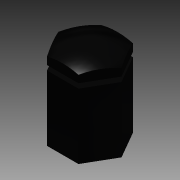
# Autodesk Inventor part: Tapón tornillo
Saved by Autodesk Inventor 2014 (Build 180170000, 170)
## iProperties
Created: 2015-05-28
Part Number: Tapón tornillo
Material: Generic
Document SubType Name: Modeling
Designer: Rubén
Density: 1 g/cm^3
Appearance: Smooth - Black
Author: Rubén
Autodesk Inventor part; units mm, degrees
ref_plane "YZ Plane" through (0, 0, 0) normal (1, 0, 0) x (0, 1, 0)
sketch "Sketch1" plane through (0, 0, 0) normal (0, 1, 0) x (-1, 0, 0)
  circle A0 centre (0, 0) radius 10.25 construction
  line L0 (5.9178, 10.25) -> (11.8357, 0)
  line L1 (11.8357, 0) -> (5.9178, -10.25)
  line L2 (5.9178, -10.25) -> (-5.9178, -10.25)
  line L3 (-5.9178, -10.25) -> (-11.8357, 0)
  line L4 (-11.8357, 0) -> (-5.9178, 10.25)
  line L5 (-5.9178, 10.25) -> (5.9178, 10.25)
  line L6 (0, 0) -> (13.5662, 0) construction
  point P0 (0, 10.25)
  dimension "d1" = 20.5
  constraints: 14 end point, 2 coincident, 1 horizontal, 1 midpoint, 1 parallel, 1 vertical alignment, 15 other
extrude "Extrusion1" add sketch "Sketch1" along normal blind 32
ref_plane "Work Plane1" through (0, 24.5, 0) normal (0, -1, 0) x (1, 0, 0)
sketch "Sketch2" plane through (0, 24.5, 0) normal (0, -1, 0) x (1, 0, 0)
  circle A0 centre (0, 0) radius 7.5 construction
  line L0 (-4.3301, 7.5) -> (4.3301, 7.5)
  line L1 (4.3301, 7.5) -> (8.6603, 0)
  line L2 (8.6603, 0) -> (4.3301, -7.5)
  line L3 (4.3301, -7.5) -> (-4.3301, -7.5)
  line L4 (-4.3301, -7.5) -> (-8.6603, 0)
  line L5 (-8.6603, 0) -> (-4.3301, 7.5)
  line L6 (0, 0) -> (-12.4427, 0) construction
  circle A1 centre (0, 0) radius 12.5
  point P0 (-6.4952, 3.75)
  dimension "d5" = 15
  dimension "d6" = 25
  constraints: 14 end point, 3 coincident, 1 centre point, 1 horizontal, 1 midpoint, 1 parallel, 16 other
  measures "d6" diameter of A1
extrude "Extrusion2" cut sketch "Sketch2" against normal blind 1.8
ref_plane "Work Plane2" through (0, 32, 10.25) normal (1, 0, 0) x (0, 1, 0)
sketch "Sketch3" plane through (0, 32, 10.25) normal (1, 0, 0) x (0, 1, 0)
  line L0 (0, 0) -> (0, -10.25)
  line L1 (-2.2, 2.6994) -> (-2.2, -15.47) construction
  line L2 (0, -10.25) -> (-2.2, -10.25) construction
  line L3 (0, 0) -> (-2.2, 0) construction
  line L4 (0, -20.5) -> (0, -10.25)
  line L5 (0, -20.5) -> (-2.2, -20.5)
  arc A0 (-2.2, -20.5) -> (-4.9254, 4.6427) centre (-24.9778, -10.25) ccw
  line L6 (0, 0) -> (0, 4.6427)
  line L7 (0, 4.6427) -> (-4.9254, 4.6427)
  point P0 (-32, -10.25)
  constraints: 16 end point, 4 point on circle, 3 perpendicular, 2 parallel, 2 point on line, 2 symmetric about line, 1 centre point, 1 vertical
revolve "Revolution1" cut sketch "Sketch3" angle 360 about axis through (0, 32, 0) along (0, -1, 0) contours L0 A0 L7 L6
sketch "Sketch4" plane through (0, 0, 0) normal (0, -1, 0) x (1, 0, 0)
  line L0 (11.8357, 0) -> (5.9178, 10.25) projected
  line L1 (-5.9178, 10.25) -> (0, 0) construction
  line L2 (-4.9075, 8.5) -> (4.9075, 8.5)
  line L3 (4.9075, 8.5) -> (9.815, 0)
  line L4 (9.815, 0) -> (4.9075, -8.5)
  line L5 (4.9075, -8.5) -> (-4.9075, -8.5)
  line L6 (-4.9075, -8.5) -> (-9.815, 0)
  line L7 (-9.815, 0) -> (-4.9075, 8.5)
  dimension "d12" = 17
  constraints: 14 end point, 1 coincident, 1 parallel, 1 point on line, 13 other
  measures "d12" distance between parallel lines of L5 L2
extrude "Extrusion3" cut sketch "Sketch4" against normal blind 22.8
body "Solid1"
